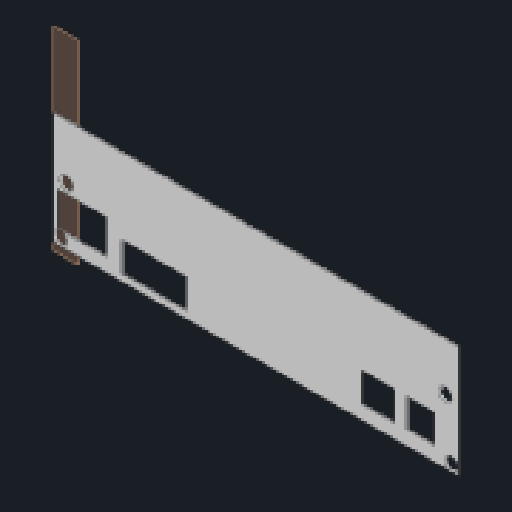
# Autodesk Inventor part: ceil_front
Saved by Autodesk Inventor 2023 (Build 270158000, 158)
## iProperties
Created: 2024-04-28
Part Number: ceil_front
Material: ABS Plastic
Document SubType Name: Modeling
Designer: szymo
Density: 1.06 g/cm^3
Appearance: Smooth - White
Mass: 16.2132 g
Surface Area: 168.318 cm^2
Volume: 15.2955 cm^3
Author: szymo
Autodesk Inventor part; units mm, degrees
ref_plane "YZ Plane" through (0, 0, 0) normal (1, 0, 0) x (0, 1, 0)
ref_plane "XZ Plane" through (0, 0, 0) normal (0, 1, 0) x (-1, 0, 0)
ref_plane "XY Plane" through (0, 0, 0) normal (0, 0, 1) x (1, 0, 0)
ref_plane "Work Plane1" through (0, 0, 0) normal (0, 0, 1) x (1, 0, 0)
sketch "Sketch1" plane through (0, 0, 0) normal (0, 0, 1) x (1, 0, 0)
  circle A0 centre (118.7, -21.5445) radius 2.5 projected
  circle A1 centre (113.95, -8.8843) radius 2.5 projected
  circle A2 centre (64.05, -19.8657) radius 2.5 projected
  circle A3 centre (59.3, -7.2055) radius 2.5 projected
  circle A4 centre (64.05, -8.8843) radius 2.5 projected
  circle A5 centre (59.3, -21.5445) radius 2.5 projected
  circle A6 centre (118.7, -7.2055) radius 2.5 projected
  circle A7 centre (113.95, -19.8657) radius 2.5 projected
  line L0 (84.5, 12.4325) -> (84.5, -11.5675) projected
  line L1 (84.5, -11.5675) -> (72.5, -11.5675) projected
  line L2 (72.5, -11.5675) -> (72.5, 4.5875) projected
  circle A8 centre (69.5, 4.5875) radius 3 projected
  line L3 (72.5, 4.5875) -> (72.5, 12.4325) projected
  line L4 (72.5, 12.4325) -> (84.5, 12.4325) projected
  arc A9 (105.5, 4.2836) -> (105.5, 4.8914) centre (108.4846, 4.5875) ccw projected
  line L5 (105.5, 4.2836) -> (105.5, -11.5675) projected
  line L6 (105.5, -11.5675) -> (93.5, -11.5675) projected
  line L7 (93.5, -11.5675) -> (93.5, 12.4325) projected
  line L8 (93.5, 12.4325) -> (105.5, 12.4325) projected
  line L9 (105.5, 12.4325) -> (105.5, 4.8914) projected
  circle A10 centre (108.4462, 27.5) radius 3 projected
  circle A11 centre (69.5, 27.5) radius 3 projected
  circle A12 centre (89, 0.9661) radius 3 projected
  circle A13 centre (89, 29.5) radius 3 projected
  arc A14 (175, 0) -> (178, -3) centre (175, -3) ccw projected
  line L10 (175, 0) -> (112.5, 0) projected
  line L11 (65.5, 33.8) -> (65.5, 0) projected
  line L12 (65.5, 0) -> (3, 0) projected
  arc A15 (0, -3) -> (3, 0) centre (3, -3) ccw projected
  line L13 (0, -3) -> (0, -25.75) projected
  arc A16 (3, -28.75) -> (0, -25.75) centre (3, -25.75) ccw projected
  line L14 (3, -28.75) -> (175, -28.75) projected
  arc A17 (178, -25.75) -> (175, -28.75) centre (175, -25.75) ccw projected
  line L15 (178, -25.75) -> (178, -3) projected
  circle A18 centre (3, -25.75) radius 2.3 projected
  circle A19 centre (3, -3) radius 2.3 projected
  circle A20 centre (3, -74.8889) radius 2.3 projected
  line L16 (0, 0) -> (6, 0) projected
  line L17 (0, -77.8889) -> (0, 0) projected
  line L18 (0, -77.8889) -> (6, -77.8889) projected
  line L19 (6, -71.8889) -> (6, -77.8889) projected
  line L20 (6, -71.8889) -> (1.6, -71.8889) projected
  line L21 (1.6, -71.8889) -> (1.6, -56.7889) projected
  line L22 (1.6, -56.7889) -> (9.6, -56.7889) projected
  line L23 (9.6, -44.7889) -> (9.6, -56.7889) projected
  line L24 (3, -44.7889) -> (9.6, -44.7889) projected
  line L25 (3, -28.75) -> (3, -44.7889) projected
  line L26 (3, -28.75) -> (6, -28.75) projected
  line L27 (6, -28.75) -> (6, -22.75) projected
  line L28 (6, -22.75) -> (3, -22.75) projected
  line L29 (3, -6) -> (3, -22.75) projected
  line L30 (3, -6) -> (6, -6) projected
  line L31 (6, -6) -> (6, 0) projected
  circle A21 centre (5.6, -52.7889) radius 2.6 projected
  circle A22 centre (175, -3) radius 2.3 projected
  circle A23 centre (175, -25.75) radius 2.3 projected
  line L32 (175, -28.75) -> (175, -41.8889) projected
  line L33 (168.4, -41.8889) -> (175, -41.8889) projected
  line L34 (168.4, -53.8889) -> (168.4, -41.8889) projected
  line L35 (175, -53.8889) -> (168.4, -53.8889) projected
  line L36 (175, -53.8889) -> (175, -71.8889) projected
  line L37 (175, -71.8889) -> (172, -71.8889) projected
  line L38 (172, -71.8889) -> (172, -77.8889) projected
  line L39 (178, -77.8889) -> (172, -77.8889) projected
  line L40 (178, -77.8889) -> (178, 0) projected
  line L41 (178, 0) -> (172, 0) projected
  line L42 (172, 0) -> (172, -6) projected
  line L43 (172, -6) -> (175, -6) projected
  line L44 (175, -6) -> (175, -22.75) projected
  line L45 (175, -22.75) -> (172, -22.75) projected
  line L46 (172, -22.75) -> (172, -28.75) projected
  line L47 (172, -28.75) -> (175, -28.75) projected
  circle A24 centre (175, -74.8889) radius 2.3 projected
  circle A25 centre (172.4, -49.8889) radius 2.6 projected
  line L48 (156.2, -70.4889) -> (156.2, -59.9889) projected
  line L49 (166.7, -59.9889) -> (156.2, -59.9889) projected
  line L50 (166.7, -59.9889) -> (166.7, -70.4889) projected
  line L51 (156.2, -70.4889) -> (166.7, -70.4889) projected
  line L52 (149, -59.8889) -> (149, -70.8889) projected
  line L53 (149, -70.8889) -> (136.35, -70.8889) projected
  line L54 (136.35, -70.8889) -> (136.35, -59.8889) projected
  line L55 (136.35, -59.8889) -> (149, -59.8889) projected
  line L56 (135, -53.8889) -> (135, -71.8889) projected
  line L57 (135, -71.8889) -> (175, -71.8889) projected
  line L58 (175, -71.8889) -> (175, -53.8889) projected
  line L59 (175, -53.8889) -> (135, -53.8889) projected
  circle A26 centre (137.85, -56.7389) radius 1.5 projected
  circle A27 centre (172.15, -56.7389) radius 1.5 projected
  line L60 (31.25, -62.8889) -> (31.25, -73.8889) projected
  line L61 (31.25, -73.8889) -> (57.25, -73.8889) projected
  line L62 (57.25, -73.8889) -> (57.25, -62.8889) projected
  line L63 (57.25, -62.8889) -> (31.25, -62.8889) projected
  line L64 (9.6, -56.7889) -> (23.3, -56.7889) projected
  line L65 (23.3, -56.7889) -> (23.3, -59.8889) projected
  line L66 (23.3, -59.8889) -> (23.3, -65.1889) projected
  line L67 (3, -71.8889) -> (23.3, -71.8889) projected
  line L68 (23.3, -61.8889) -> (23.3, -74.8889) projected
  line L69 (30.25, -61.8889) -> (30.25, -74.8889)
  line L70 (30.25, -74.8889) -> (58.25, -74.8889)
  line L71 (58.25, -74.8889) -> (58.25, -61.8889)
  line L72 (58.25, -61.8889) -> (30.25, -61.8889)
  line L73 (150, -58.8889) -> (150, -71.8889)
  line L74 (150, -71.8889) -> (135.35, -71.8889)
  line L75 (135.35, -71.8889) -> (135.35, -58.8889)
  line L76 (135.35, -58.8889) -> (150, -58.8889)
  line L77 (155.2, -58.9889) -> (155.2, -71.4889)
  line L78 (155.2, -71.4889) -> (167.7, -71.4889)
  line L79 (167.7, -71.4889) -> (167.7, -58.9889)
  line L80 (167.7, -58.9889) -> (155.2, -58.9889)
  line L81 (0, -28.75) -> (178, -28.75)
  line L82 (178, -28.75) -> (178, -77.8889)
  line L83 (178, -77.8889) -> (0, -77.8889)
  line L84 (0, -77.8889) -> (0, -28.75)
  line L85 (131.125, -21.1625) -> (131.125, -7.525) projected
  arc A28 (134.125, -4.525) -> (131.125, -7.525) centre (134.125, -7.525) ccw projected
  line L86 (134.125, -4.525) -> (155.95, -4.525) projected
  arc A29 (158.95, -7.525) -> (155.95, -4.525) centre (155.95, -7.525) ccw projected
  line L87 (158.95, -7.525) -> (158.95, -21.1625) projected
  arc A30 (155.95, -24.1625) -> (158.95, -21.1625) centre (155.95, -21.1625) ccw projected
  line L88 (155.95, -24.1625) -> (134.125, -24.1625) projected
  arc A31 (131.125, -21.1625) -> (134.125, -24.1625) centre (134.125, -21.1625) ccw projected
  line L89 (46.875, -7.5875) -> (46.875, -21.225) projected
  arc A32 (43.875, -24.225) -> (46.875, -21.225) centre (43.875, -21.225) ccw projected
  line L90 (43.875, -24.225) -> (22.05, -24.225) projected
  arc A33 (19.05, -21.225) -> (22.05, -24.225) centre (22.05, -21.225) ccw projected
  line L91 (19.05, -21.225) -> (19.05, -7.5875) projected
  arc A34 (22.05, -4.5875) -> (19.05, -7.5875) centre (22.05, -7.5875) ccw projected
  line L92 (22.05, -4.5875) -> (43.875, -4.5875) projected
  arc A35 (46.875, -7.5875) -> (43.875, -4.5875) centre (43.875, -7.5875) ccw projected
  line L93 (112.5, 0) -> (112.5, 33.8) projected
  line L94 (112.5, 33.8) -> (65.5, 33.8) projected
  point P0 (3, -28.75)
  point P1 (175, -28.75)
  point P2 (135.35, -71.8889)
  dimension "d0" = 1
  dimension "d1" = 1
  dimension "d2" = 1
  constraints: 32 end point, 2 parallel, 1 horizontal, 1 horizontal alignment, 1 perpendicular, 1 point on line, 9 other
  measures "d0" distance between parallel lines of L63 L72
  measures "d1" distance between parallel lines of L55 L76
  measures "d2" distance between parallel lines of L49 L80
extrude "Extrusion1" add sketch "Sketch1" along normal blind 0.6 contours L40 L39 L38 L37 L36 L35 L34 L33 L32 L81 | L32 L33 L34 L59 L56 L57 L38 L83 L19 L67 L68 L66 L65 L64 L23 L24 L25 L14 | L25 L24 L23 L22 L21 L20 L19 L18 L17 L81 | L57 L73 L76 L75 L56 L59 L35 L36 L37 | A20 | A21 | A24 | A25 | A26 | A27
sketch "Sketch2" plane through (0, 0, 0.6) normal (0, 0, 1) x (1, 0, 0)
  circle A0 centre (3, -25.75) radius 2.3 projected
  circle A1 centre (3, -3) radius 2.3 projected
  circle A2 centre (3, -74.8889) radius 2.3 projected
  line L0 (0, 0) -> (6, 0) projected
  line L1 (0, -77.8889) -> (0, 0) projected
  line L2 (0, -77.8889) -> (6, -77.8889) projected
  line L3 (6, -71.8889) -> (6, -77.8889) projected
  line L4 (6, -71.8889) -> (1.6, -71.8889) projected
  line L5 (1.6, -71.8889) -> (1.6, -56.7889) projected
  line L6 (1.6, -56.7889) -> (9.6, -56.7889) projected
  line L7 (9.6, -44.7889) -> (9.6, -56.7889) projected
  line L8 (3, -44.7889) -> (9.6, -44.7889) projected
  line L9 (3, -28.75) -> (3, -44.7889) projected
  line L10 (3, -28.75) -> (6, -28.75) projected
  line L11 (6, -28.75) -> (6, -22.75) projected
  line L12 (6, -22.75) -> (3, -22.75) projected
  line L13 (3, -6) -> (3, -22.75) projected
  line L14 (3, -6) -> (6, -6) projected
  line L15 (6, -6) -> (6, 0) projected
  circle A3 centre (5.6, -52.7889) radius 2.6 projected
  circle A4 centre (172.4, -49.8889) radius 2.6 projected
  circle A5 centre (175, -3) radius 2.3 projected
  circle A6 centre (175, -25.75) radius 2.3 projected
  line L16 (175, -28.75) -> (175, -41.8889) projected
  line L17 (168.4, -41.8889) -> (175, -41.8889) projected
  line L18 (168.4, -53.8889) -> (168.4, -41.8889) projected
  line L19 (175, -53.8889) -> (168.4, -53.8889) projected
  line L20 (175, -53.8889) -> (175, -71.8889) projected
  line L21 (175, -71.8889) -> (172, -71.8889) projected
  line L22 (172, -71.8889) -> (172, -77.8889) projected
  line L23 (178, -77.8889) -> (172, -77.8889) projected
  line L24 (178, -77.8889) -> (178, 0) projected
  line L25 (178, 0) -> (172, 0) projected
  line L26 (172, 0) -> (172, -6) projected
  line L27 (172, -6) -> (175, -6) projected
  line L28 (175, -6) -> (175, -22.75) projected
  line L29 (175, -22.75) -> (172, -22.75) projected
  line L30 (172, -22.75) -> (172, -28.75) projected
  line L31 (172, -28.75) -> (175, -28.75) projected
  circle A7 centre (175, -74.8889) radius 2.3 projected
  circle A8 centre (172.4, -49.8889) radius 2.6 projected
  constraints: 4 coincident
hole "Hole1" at (5.6, -52.7889, 0.6) at (3, -74.8889, 0.6) at (175, -74.8889, 0.6) at (172.4, -49.8889, 0.6) direction (0, 0, -1) diameter 3.6 end through all countersink diameter 6 countersink angle 90 clearance for "Countersunk Flat Head Screw ISO 2009/7046" size "M3" standard "ISO"
body "Solid1"
